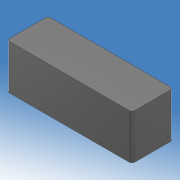
# Autodesk Inventor part: MaxAmps_battery
Saved by Autodesk Inventor 2020 (Build 240168000, 168)
## iProperties
Created: 2019-12-04
Part Number: MaxAmps_battery
Material: Generic
Document SubType Name: Modeling
Designer: mpark
Density: 1 g/cm^3
Appearance: Smooth - Black
Author: mpark
Autodesk Inventor part; units mm, degrees
ref_plane "YZ Plane" through (0, 0, 0) normal (1, 0, 0) x (0, 1, 0)
ref_plane "XZ Plane" through (0, 0, 0) normal (0, 1, 0) x (-1, 0, 0)
ref_plane "XY Plane" through (0, 0, 0) normal (0, 0, 1) x (1, 0, 0)
sketch "Sketch1" plane through (0, 0, 0) normal (0, 1, 0) x (-1, 0, 0)
  line L0 (68.5, -22.5) -> (-68.5, -22.5)
  line L1 (-68.5, -22.5) -> (-68.5, 22.5)
  line L2 (-68.5, 22.5) -> (68.5, 22.5)
  line L3 (68.5, 22.5) -> (68.5, -22.5)
  line L4 (68.5, -22.5) -> (-68.5, 22.5) construction
  line L5 (-68.5, -22.5) -> (68.5, 22.5) construction
  point P0 (0, 0)
  dimension "d0" = 137
  dimension "d1" = 45
  constraints: 12 end point, 2 midpoint, 2 parallel, 1 horizontal, 1 perpendicular
  measures "d0" distance of L1.end L2.end
  measures "d1" distance of L0.end L1.end
extrude "Extrusion1" add sketch "Sketch1" along normal blind 49
fillet "Fillet1" radius 3 4 edges at (-68.5, 24.5, 22.5) (-68.5, 24.5, -22.5) (68.5, 24.5, -22.5) (68.5, 24.5, 22.5)
body "Solid1"
